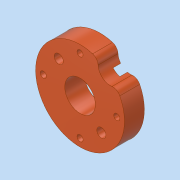
# Autodesk Inventor part: idlerShaftBearingMount
Saved by Autodesk Inventor 2017 (Build 210142000, 142)
## iProperties
Created: 2016-11-30
Part Number: idlerShaftBearingMount
Material: ABS Plastic
Document SubType Name: Modeling
Designer: techn
Density: 1.06 g/cm^3
Appearance: Smooth - Light Orange
Author: techn
Autodesk Inventor part; units mm, degrees
ref_plane "YZ Plane" through (0, 0, 0) normal (1, 0, 0) x (0, 1, 0)
ref_plane "XZ Plane" through (0, 0, 0) normal (0, 1, 0) x (-1, 0, 0)
ref_plane "XY Plane" through (0, 0, 0) normal (0, 0, 1) x (1, 0, 0)
sketch "Sketch7" plane through (0, 0, 0) normal (0, 0, 1) x (1, 0, 0)
  line L0 (0, 0) -> (0, 15.24)
  circle A0 centre (0, 15.24) radius 1.27
  circle A1 centre (-15.24, 0) radius 1.27
  circle A2 centre (0, -15.24) radius 1.27
  circle A3 centre (15.24, 0) radius 1.27
  circle A4 centre (0, 0) radius 18.415
  line L1 (0, 0) -> (8.4414, 8.4414)
  line L2 (0, 0) -> (11.938, 0) construction
  circle A5 centre (8.4414, 8.4414) radius 3.3655
  dimension "d82" = 15.24
  dimension "d83" = 2.54
  dimension "d86" = 360
  dimension "d88" = 36.83
  dimension "d89" = 11.938
  dimension "d90" = 45
  dimension "d91" = 6.731
  constraints: 6 centre point, 6 end point, 3 coincident, 1 equal length, 1 horizontal, 1 vertical, 9 other
  measures "d82" distance of L0.start L0.end
  measures "d83" diameter of A0
  measures "d88" diameter of A4
  measures "d89" distance of L1.start L1.end
  measures "d90" angle of L2 L1
  measures "d91" diameter of A5
extrude "Extrusion8" add sketch "Sketch7" along normal blind 8.255
sketch "Sketch8" plane through (0, 0, 8.255) normal (0, 0, 1) x (1, 0, 0)
  circle A0 centre (0, 0) radius 6.35
  dimension "d94" = 12.7
  constraints: 1 centre point, 1 coincident
  measures "d94" diameter of A0
extrude "Extrusion9" cut sketch "Sketch8" against normal through all
sketch "Sketch10" plane through (0, 0, 8.255) normal (0, 0, 1) x (1, 0, 0)
  circle A0 centre (8.4414, 8.4414) radius 3.3655 projected
  point P0 (0, 0)
extrude "Extrusion10" add sketch "Sketch10" against normal blind 5.08
sketch "Sketch11" plane through (0, 0, 8.255) normal (0, 0, 1) x (1, 0, 0)
  line L0 (0, 0) -> (-8.8388, 8.8388)
  line L1 (0, 0) -> (12.5, 0) construction
  line L2 (0, 0) -> (8.8388, -8.8388)
  circle A0 centre (-8.8388, 8.8388) radius 1.905
  circle A1 centre (8.8388, -8.8388) radius 1.905
  dimension "d99" = 12.5
  dimension "d100" = 135
  dimension "d101" = 12.5
  dimension "d102" = 3.81
  dimension "d103" = 3.81
  constraints: 6 end point, 2 centre point, 2 coincident, 1 collinear, 1 equal length, 1 horizontal
  measures "d99" distance of L0.start L0.end
  measures "d100" angle of L1 L0
  measures "d101" distance of L0.start L2.end
  measures "d102" diameter of A0
  measures "d103" diameter of A1
extrude "Extrusion11" cut sketch "Sketch11" against normal through all
sketch "Sketch12" plane through (0, 0, 0) normal (0, 0, -1) x (-1, 0, 0)
  circle A0 centre (0, 0) radius 6.3532
  constraints: 1 centre point, 1 coincident
extrude "Extrusion12" cut sketch "Sketch12" against normal through all
sketch "Sketch13" plane through (0, 0, 0) normal (0, 0, -1) x (-1, 0, 0)
  circle A0 centre (0, 0) radius 18.415 projected
  circle A1 centre (0, 15.24) radius 1.27 projected
  circle A2 centre (15.24, 0) radius 1.27 projected
  circle A3 centre (0, -15.24) radius 1.27 projected
  circle A4 centre (-15.24, 0) radius 1.27 projected
  circle A5 centre (0, 0) radius 6.3532 projected
  circle A6 centre (-8.4414, 8.4414) radius 3.3655 projected
  circle A7 centre (-8.8388, -8.8388) radius 1.905 projected
  circle A8 centre (8.8388, 8.8388) radius 1.905 projected
  line L0 (0, 0) -> (-15.0847, 10.5624) construction
  circle A9 centre (0, 0) radius 18.415 construction
  line L1 (0, 0) -> (18.415, 0) construction
  arc A10 (-15.0847, 10.5624) -> (-7.7825, 16.6897) centre (-12.5636, 14.9727) ccw
  line L2 (-7.7825, 16.6897) -> (0, 0) construction
  arc A11 (-7.7825, 16.6897) -> (-15.0847, 10.5624) centre (0, 0) ccw
  dimension "d112" = 145
  dimension "d113" = 30
  dimension "d114" = 5.08
  constraints: 6 end point, 6 point on circle, 2 centre point, 1 equal length, 1 horizontal, 2 other
  measures "d112" angle of L1 L0
  measures "d113" angle of L0 L2
  measures "d114" radius of A10
extrude "Extrusion13" cut sketch "Sketch13" against normal through all contours A10 A6 A0 | A10 A6 picked at (-11.1725, 13.188) picked at (-10.0868, 10.8311)
fillet "Fillet4" radius 3.175 2 edges at (7.7825, 16.6897, 4.1275) (15.0847, 10.5624, 4.1275)
equation "\"d101\" = d99"
equation "\"d102\" = d103"
body "Solid3"
